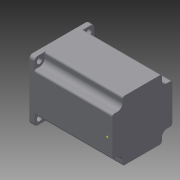
# Autodesk Inventor part: G723-280-4
Saved by Autodesk Inventor 2013 (Build 170138000, 138)
## iProperties
Created: 2012-11-28
Part Number: G723-280-4
Material: Generic
Document SubType Name: Modeling
Designer: istvan.burbank
Density: 1 g/cm^3
Mass: 258.816 g
Surface Area: 246.452 cm^2
Volume: 258.816 cm^3
Author: istvan.burbank
Autodesk Inventor part; units mm, degrees
ref_plane "YZ Plane" through (0, 0, 0) normal (1, 0, 0) x (0, 1, 0)
ref_plane "XZ Plane" through (0, 0, 0) normal (0, 1, 0) x (-1, 0, 0)
ref_plane "XY Plane" through (0, 0, 0) normal (0, 0, 1) x (1, 0, 0)
sketch "Sketch1" plane through (0, 0, 0) normal (1, 0, 0) x (0, 1, 0)
  line L0 (3.175, 0) -> (53.975, 0)
  line L1 (57.15, 3.175) -> (57.15, 53.975)
  line L2 (53.975, 57.15) -> (3.175, 57.15)
  line L3 (0, 53.975) -> (0, 3.175)
  arc A0 (3.175, 57.15) -> (0, 53.975) centre (3.175, 53.975) ccw
  arc A1 (57.15, 53.975) -> (53.975, 57.15) centre (53.975, 53.975) ccw
  arc A2 (53.975, 0) -> (57.15, 3.175) centre (53.975, 3.175) ccw
  arc A3 (0, 3.175) -> (3.175, 0) centre (3.175, 3.175) ccw
  point P0 (0, 0)
  point P1 (57.15, 57.15)
  point P2 (57.15, 0)
  point P3 (0, 57.15)
  dimension "d0" = 57.15
  dimension "d1" = 57.15
  dimension "d17" = 3.175
  constraints: 8 end point, 8 point on circle, 8 point on line, 8 tangent, 4 centre point, 3 equal radius, 2 parallel, 1 horizontal, 1 perpendicular
  measures "d0" distance of point (0, 57.15) point (57.15, 57.15)
  measures "d1" distance of point (57.15, 57.15) point (57.15, 0)
  measures "d17" radius of A0
extrude "Extrusion1" add sketch "Sketch1" along normal blind 78.74
sketch "Sketch2" plane through (0, 0, 0) normal (-1, 0, 0) x (0, 0, 1)
  line L0 (0, 53.975) -> (0, 3.175) projected
  line L1 (53.975, 57.15) -> (3.175, 57.15) projected
  circle A0 centre (28.575, 28.575) radius 19.05
  point P0 (0, 57.15)
  point P1 (0, 0)
  point P2 (57.15, 57.15)
  dimension "d4" = 38.1
  dimension "d18" = 28.575
  dimension "d19" = 28.575
  constraints: 1 centre point
  measures "d4" diameter of A0
  measures "d18" distance from line of L1 A0.centre
  measures "d19" distance from line of L0 A0.centre
extrude "Extrusion2" add sketch "Sketch2" along normal blind 1.524
sketch "Sketch3" plane through (-1.524, 28.575, 28.575) normal (-1, 0, 0) x (0, 0, 1)
  circle A0 centre (0, 0) radius 19.05 projected
  circle A1 centre (0, 0) radius 3.175
  point P0 (-28.575, -28.575)
  dimension "d10" = 6.35
  constraints: 1 centre point, 1 coincident
  measures "d10" diameter of A1
extrude "Extrusion3" add sketch "Sketch3" along normal blind 19.05 contours A1
sketch "Sketch4" plane through (-20.574, 28.575, 28.575) normal (-1, 0, 0) x (0, 0, 1)
  circle A0 centre (0, 0) radius 3.175 projected
  line L0 (-1.7227, 2.667) -> (1.7227, 2.667)
  line L1 (0, -3.175) -> (-5.2914, -3.175)
  point P0 (-28.575, -28.575)
  dimension "d13" = 5.842
  constraints: 4 end point, 3 point on circle, 1 horizontal, 1 parallel, 1 tangent
  measures "d13" distance between parallel lines of L0 L1
extrude "Extrusion4" cut sketch "Sketch4" against normal blind 14.986 contours L0 A0 picked at (-0.1211, 2.8294)
sketch "Sketch5" plane through (78.74, 0, 0) normal (1, 0, 0) x (0, 0, -1)
  line L0 (-57.15, 53.975) -> (-57.15, 3.175) projected
  arc A0 (-57.15, 3.175) -> (-53.975, 0) centre (-53.975, 3.175) ccw projected
  line L1 (-53.975, 0) -> (-3.175, 0) projected
  arc A1 (-3.175, 0) -> (0, 3.175) centre (-3.175, 3.175) ccw projected
  line L2 (0, 3.175) -> (0, 53.975) projected
  arc A2 (0, 53.975) -> (-3.175, 57.15) centre (-3.175, 53.975) ccw projected
  line L3 (-3.175, 57.15) -> (-53.975, 57.15) projected
  arc A3 (-53.975, 57.15) -> (-57.15, 53.975) centre (-53.975, 53.975) ccw projected
  circle A4 centre (-52.197, 52.197) radius 2.54
  circle A5 centre (-52.197, 52.197) radius 4.953
  line L4 (-3.175, 57.15) -> (-53.975, 57.15) projected
  line L5 (-52.197, 47.244) -> (-57.15, 47.244)
  line L6 (-57.15, 47.244) -> (-57.15, 57.15)
  line L7 (-57.15, 57.15) -> (-47.244, 57.15)
  line L8 (-47.244, 57.15) -> (-47.244, 52.197)
  circle A6 centre (-4.953, 52.197) radius 4.953
  circle A7 centre (-4.953, 4.953) radius 4.953
  circle A8 centre (-52.197, 4.953) radius 4.953
  line L9 (0, 3.175) -> (0, 53.975) projected
  line L10 (-53.975, 0) -> (-3.175, 0) projected
  line L11 (-57.15, 53.975) -> (-57.15, 3.175) projected
  line L12 (0, 57.15) -> (-9.906, 57.15)
  line L13 (-9.906, 57.15) -> (-9.906, 52.197)
  line L14 (-4.953, 47.244) -> (0, 47.244)
  line L15 (0, 47.244) -> (0, 57.15)
  line L16 (-57.15, 0) -> (-47.244, 0)
  line L17 (-47.244, 0) -> (-47.244, 4.953)
  line L18 (-52.197, 9.906) -> (-57.15, 9.906)
  line L19 (-57.15, 9.906) -> (-57.15, 0)
  line L20 (-4.953, 9.906) -> (0, 9.906)
  line L21 (0, 9.906) -> (0, 0)
  line L22 (0, 0) -> (-9.906, 0)
  line L23 (-9.906, 0) -> (-9.906, 4.953)
  dimension "d48" = 4.953
  dimension "d49" = 4.953
  dimension "d50" = 5.08
  dimension "d51" = 9.906
  dimension "d52" = 9.906
  dimension "d53" = 9.906
  dimension "d54" = 9.906
  dimension "d55" = 9.906
  dimension "d56" = 9.906
  dimension "d57" = 9.906
  dimension "d58" = 9.906
  dimension "d59" = 9.906
  dimension "d60" = 9.906
  dimension "d61" = 9.906
  dimension "d62" = 9.906
  dimension "d63" = 9.906
  constraints: 32 end point, 8 parallel, 8 point on circle, 7 tangent, 5 centre point, 4 horizontal, 4 perpendicular, 2 coincident
  measures "d48" distance from line of L0 point (-52.197, 52.197)
  measures "d49" distance from line of L3 point (-52.197, 52.197)
  measures "d50" diameter of A4
  measures "d51" diameter of A8
  measures "d52" diameter of A7
  measures "d53" diameter of A6
  measures "d54" distance between parallel lines of L2 L23
  measures "d55" distance between parallel lines of L1 L20
  measures "d56" distance between parallel lines of L2 L13
  measures "d57" distance between parallel lines of L3 L14
  measures "d58" distance between parallel lines of L0 L8
  measures "d59" distance between parallel lines of L4 L5
  measures "d60" distance between parallel lines of L0 L17
  measures "d61" distance between parallel lines of L1 L18
  measures "d62" distance between parallel lines of L14 L12
  measures "d63" distance between parallel lines of L5 L3
extrude "Extrusion6" cut sketch "Sketch5" against normal blind 74.041 contours L0 A5 L5 | L18 A8 L0 | L0 A3 L3 A5 | A5 | A8 L1 A0 L0 | A8 | L6 L7 A3 | L3 L8 A5 | A0 L16 L19 | A8 L17 L1 | L3 A6 L13 | L23 A7 L1 | L3 A2 L2 A6 | A6 | A7 L2 A1 L1 | A7 | L12 L15 A2 | L2 L14 A6 | A1 L21 L22 | A7 L20 L2 | A4
fillet "Fillet1" radius 1.905 8 edges at (41.7195, 57.15, 47.244) (41.7195, 47.244, 57.15) (41.7195, 57.15, 9.906) (41.7195, 47.244, 0) (41.7195, 9.906, 0) (41.7195, 0, 9.906) (41.7195, 0, 47.244) (41.7195, 9.906, 57.15)
sketch "Sketch6" plane through (0, 0, 0) normal (-1, 0, 0) x (0, 0, 1)
  line L0 (53.975, 57.15) -> (3.175, 57.15) projected
  line L1 (0, 53.975) -> (0, 3.175) projected
  point P0 (0, 0)
  point P1 (4.953, 52.197)
  point P2 (52.197, 52.197)
  point P3 (52.197, 4.953)
  point P4 (4.953, 4.953)
  dimension "d36" = 47.244
  dimension "d37" = 47.244
  dimension "d39" = 4.953
  dimension "d40" = 4.953
  constraints: 2 horizontal alignment, 2 vertical alignment
  measures "d36" distance of point (52.197, 52.197) point (4.953, 52.197)
  measures "d37" distance of point (4.953, 4.953) point (4.953, 52.197)
  measures "d39" distance from line of L1 point (4.953, 52.197)
  measures "d40" distance from line of L0 point (4.953, 52.197)
hole "Hole1" at (0, 52.197, 4.953) at (0, 52.197, 52.197) at (0, 4.953, 52.197) at (0, 4.953, 4.953) direction (1, 0, 0) diameter 5.08 end through all
body "Solid1"
